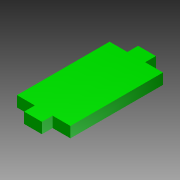
# Autodesk Inventor part: servo_holer2
Saved by Autodesk Inventor 2012 (Build 160160000, 160)
## iProperties
Created: 2013-10-02
Part Number: servo_holer2
Material: Default
Document SubType Name: Modeling
Designer: Nick
Density: 1 g/cm^3
Author: Nick
Autodesk Inventor part; units mm, degrees
ref_plane "YZ Plane" through (0, 0, 0) normal (1, 0, 0) x (0, 1, 0)
ref_plane "XZ Plane" through (0, 0, 0) normal (0, 1, 0) x (-1, 0, 0)
ref_plane "XY Plane" through (0, 0, 0) normal (0, 0, 1) x (1, 0, 0)
sketch "Sketch1" plane through (0, 0, 0) normal (0, 0, 1) x (1, 0, 0)
  line L0 (15, 0) -> (15, 26)
  line L1 (0, 26) -> (0, 0)
  line L2 (10, 26) -> (10, 29)
  line L3 (10, 29) -> (5, 29)
  line L4 (5, 29) -> (5, 26)
  line L5 (10, 0) -> (10, -3)
  line L6 (10, -3) -> (5, -3)
  line L7 (5, -3) -> (5, 0)
  line L8 (15, 26) -> (10, 26)
  line L9 (5, 26) -> (0, 26)
  line L10 (0, 0) -> (5, 0)
  line L11 (10, 0) -> (15, 0)
  point P0 (5, 27.5)
  point P1 (5, -1.5)
  dimension "d0" = 3
  dimension "d1" = 3
  dimension "d2" = 5
  dimension "d3" = 26
  dimension "d4" = 15
  dimension "d5" = 5
  constraints: 24 end point, 7 parallel, 3 horizontal alignment, 3 vertical alignment, 2 horizontal, 2 midpoint, 2 perpendicular
  measures "d0" distance of L2.start L2.end
  measures "d1" distance of L5.start L5.end
  measures "d2" distance of L2.end L3.end
  measures "d3" distance of L1.start L1.end
  measures "d4" distance between parallel lines of L1 L0
  measures "d5" distance between parallel lines of L1 L4
extrude "Extrusion1" add sketch "Sketch1" along normal blind 3
equation "\"d1\" = d0"
equation "\"d5\" = 0.5 * d4 - 0.5 * d2"
body "Solid1"
